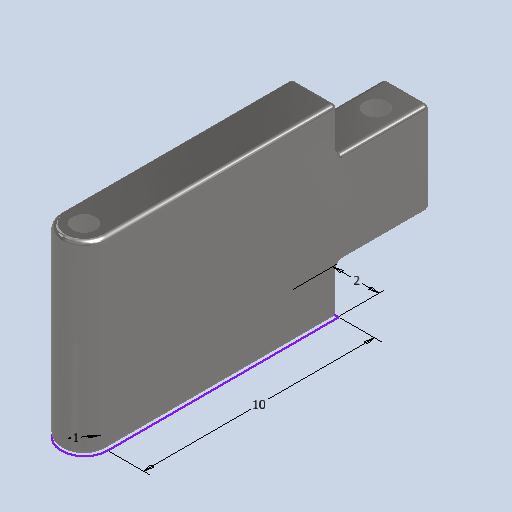
# Autodesk Inventor part: Link1
Saved by Autodesk Inventor 2022 (Build 260153000, 153)
## iProperties
Part Number: Link1
Material: Generic
Document SubType Name: Modeling
Designer: suhas
Appearance: Default
Author: suhas
Autodesk Inventor part; units mm, degrees
ref_plane "YZ Plane" through (0, 0, 0) normal (1, 0, 0) x (0, 1, 0)
ref_plane "XZ Plane" through (0, 0, 0) normal (0, 1, 0) x (-1, 0, 0)
ref_plane "XY Plane" through (0, 0, 0) normal (0, 0, 1) x (1, 0, 0)
sketch "Sketch1" plane through (0, 0, 0) normal (0, 1, 0) x (-1, 0, 0)
  arc A0 (10, 0) -> (-10, 0) centre (0, 0) ccw
  circle A1 centre (0, 0) radius 5
  line L0 (-10, 0) -> (-10, -100)
  line L1 (-10, -100) -> (10, -100)
  line L2 (10, -100) -> (10, 0)
  dimension "d1" = 10
  dimension "d2" = 100
  dimension "d12" = 20
  constraints: 6 end point, 2 centre point, 2 coincident, 2 point on circle, 1 parallel
  measures "d1" diameter of A1
  measures "d2" distance of L0.end L0.start
  measures "d12" distance between parallel lines of L0 L2
extrude "Extrusion1" add sketch "Sketch1" along normal blind 80
sketch "Sketch2" plane through (10, 0, -100) normal (0, 0, -1) x (-1, 0, 0)
  line L0 (20, 0) -> (20, 80) projected
  line L1 (0, 20) -> (20, 20)
  line L2 (20, 20) -> (20, 60)
  line L3 (20, 60) -> (0, 60)
  line L4 (0, 60) -> (0, 20)
  line L5 (0, 20) -> (20, 60) construction
  line L6 (20, 20) -> (0, 60) construction
  point P0 (10, 0)
  point P1 (10, 40)
  dimension "d5" = 40
  constraints: 12 end point, 2 midpoint, 2 parallel, 1 horizontal, 1 perpendicular, 1 point on line
  measures "d5" distance of L2.end L1.end
extrude "Extrusion2" add sketch "Sketch2" along normal blind 40
sketch "Sketch3" plane through (-10, 60, -100) normal (0, 1, 0) x (1, 0, 0)
  circle A0 centre (10, 26.3827) radius 5
  point P0 (10, -100)
  dimension "d8" = 10
  constraints: 1 centre point
  measures "d8" diameter of A0
extrude "Extrusion3" cut sketch "Sketch3" against normal blind 40
fillet "Fillet1" radius 2 22 edges at (0, 80, 10) (10, 80, -50) (-10, 80, -50) (10, 0, -50) (-10, 0, -50) (0, 0, 10) (-10, 70, -100) (0, 80, -100) (10, 70, -100) (-10, 10, -100) (10, 10, -100) (0, 0, -100) (0, 60, -100) (0, 20, -100) (10, 40, -140) (-10, 40, -140) (0, 20, -140) (10, 20, -120) (-10, 20, -120) (10, 60, -120) (-10, 60, -120) (0, 60, -140)
body "Solid1"
